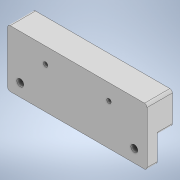
# Autodesk Inventor part: リアルセンスマウント2
Saved by Autodesk Inventor 2020 (Build 240168000, 168)
## iProperties
Created: 2019-11-22
Part Number: リアルセンスマウント2
Material: 一般
Document SubType Name: Modeling
Designer: highs
Density: 1 g/cm^3
Appearance: 既定
Author: highs
## iProperties of the stored document _3D プリント.ipt
Created: 2019-11-22
Part Number: _3D プリント
Material: 一般
Document SubType Name: Modeling
Designer: highs
Density: 1 g/cm^3
Appearance: 既定
Author: highs
Autodesk Inventor part; units mm, degrees
ref_plane "YZ Plane" through (0, 0, 0) normal (1, 0, 0) x (0, 1, 0)
ref_plane "XZ Plane" through (0, 0, 0) normal (0, 1, 0) x (-1, 0, 0)
ref_plane "XY Plane" through (0, 0, 0) normal (0, 0, 1) x (1, 0, 0)
sketch "スケッチ1" plane through (0, 0, 0) normal (0, 0, 1) x (1, 0, 0)
  line L0 (0, 0) -> (110, 0)
  line L1 (110, 0) -> (110, 45)
  line L2 (110, 45) -> (0, 45)
  line L3 (0, 45) -> (0, 0)
  line L4 (0, 32.5) -> (110, 32.5) construction
  line L5 (0, 10) -> (110, 10) construction
  circle A0 centre (10, 10) radius 2.75
  circle A1 centre (100, 10) radius 2.75
  circle A2 centre (30, 32.5) radius 1.75
  circle A3 centre (80, 32.5) radius 1.75
  line L6 (55, 45) -> (55, 0) construction
  dimension "d2" = 110
  dimension "d3" = 45
  dimension "d4" = 12.5
  dimension "d5" = 10
  dimension "d6" = 50
  dimension "d8" = 10
  dimension "d9" = 5.5
  dimension "d10" = 3.5
  constraints: 14 end point, 8 point on line, 4 centre point, 3 parallel, 2 equal radius, 2 midpoint, 2 perpendicular, 1 horizontal, 2 other
  measures "d2" distance of L0.start L0.end
  measures "d3" distance of L2.end L0.start
  measures "d4" distance between parallel lines of L2 L4
  measures "d5" distance between parallel lines of L0 L5
  measures "d6" distance of A3.centre A2.centre
  measures "d8" distance from line of L3 A0.centre
  measures "d9" diameter of A0
  measures "d10" diameter of A2
extrude "押し出し1" add sketch "スケッチ1" along normal blind 20
sketch "スケッチ2" plane through (0, 0, 0) normal (0, 0, -1) x (-1, 0, 0)
  line L0 (0, 0) -> (-110, 0) projected
  line L1 (-110, 0) -> (0, 0)
  line L2 (0, 0) -> (0, 20)
  line L3 (0, 20) -> (-110, 20)
  line L4 (-110, 20) -> (-110, 0)
  point P0 (-110, 45)
  dimension "d14" = 20
  constraints: 8 end point, 2 parallel, 1 horizontal, 1 perpendicular, 1 point on line
  measures "d14" distance between parallel lines of L0 L3
extrude "押し出し2" cut sketch "スケッチ2" against normal blind 12
fillet "フィレット1" radius 2 6 edges at (110, 0, 16) (110, 45, 10) (0, 0, 16) (0, 45, 10) (110, 20, 6) (0, 20, 6)
